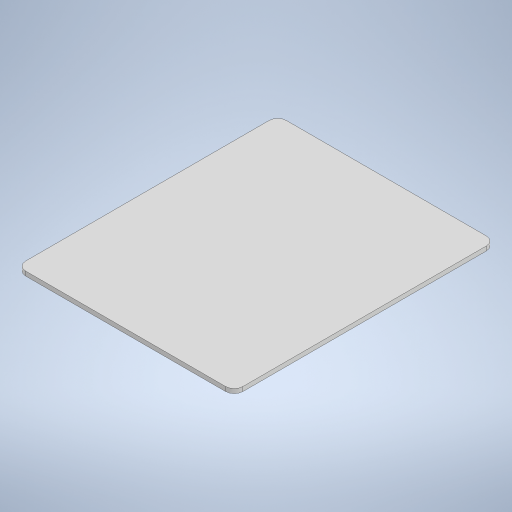
# Autodesk Inventor part: Part1
Saved by Autodesk Inventor 2024 (Build 280153000, 153)
## iProperties
Created: 2023-05-18
Part Number: Part1
Material: Generic
Document SubType Name: Modeling
Designer: shraa
Density: 1 g/cm^3
Appearance: Default
Author: shraa
Autodesk Inventor part; units mm, degrees
ref_plane "YZ Plane" through (0, 0, 0) normal (1, 0, 0) x (0, 1, 0)
ref_plane "XZ Plane" through (0, 0, 0) normal (0, 1, 0) x (-1, 0, 0)
ref_plane "XY Plane" through (0, 0, 0) normal (0, 0, 1) x (1, 0, 0)
sketch "Sketch1" plane through (0, 0, 0) normal (0, 1, 0) x (-1, 0, 0)
  line L0 (0, 0) -> (250, 0)
  line L1 (250, 0) -> (250, -300)
  line L2 (250, -300) -> (0, -300)
  line L3 (0, -300) -> (0, 0)
  dimension "d0" = 250
  dimension "d1" = 300
  constraints: 8 end point, 2 parallel, 1 horizontal, 1 perpendicular
  measures "d0" distance of L1.end L2.end
  measures "d1" distance of L0.end L1.end
extrude "Extrusion1" add sketch "Sketch1" along normal blind 5
fillet "Fillet1" radius 10 1 edges at (-250, 2.5, 0)
fillet "Fillet2" radius 10 3 edges at (0, 2.5, 0) (0, 2.5, -300) (-250, 2.5, -300)
body "Solid1"
